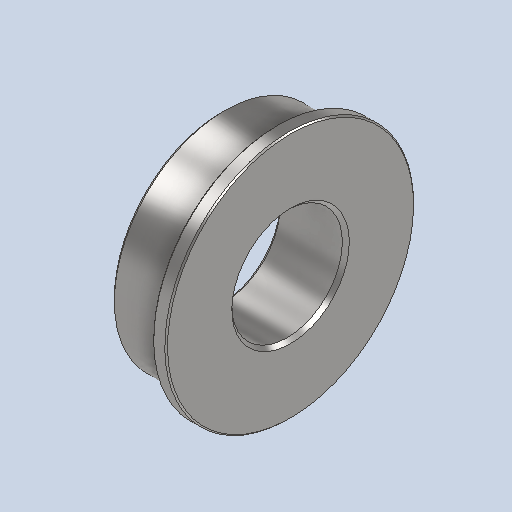
# Autodesk Inventor part: F688ZZ_V1
Saved by Autodesk Inventor 2023 (Build 270158000, 158)
## iProperties
Created: 2023-02-13
Part Number: F688ZZ_V1
Material: Stahl, Legierung
Document SubType Name: Modeling
Designer: Mathi
Density: 7.73 g/cm^3
Appearance: Halbpoliert
Author: Mathi
Autodesk Inventor part; units mm, degrees
ref_plane "YZ Plane" through (0, 0, 0) normal (1, 0, 0) x (0, 1, 0)
ref_plane "XZ Plane" through (0, 0, 0) normal (0, 1, 0) x (-1, 0, 0)
ref_plane "XY Plane" through (0, 0, 0) normal (0, 0, 1) x (1, 0, 0)
sketch "Skizze1" plane through (0, 0, 0) normal (0, 0, 1) x (1, 0, 0)
  line L0 (-18.8104, 0) -> (17.0467, 0)
  line L1 (-3.75, 4) -> (0.75, 4)
  line L2 (1, 4.25) -> (1, 8.9)
  line L3 (0.9, 9) -> (0.1, 9)
  line L4 (0, 8.9) -> (0, 8)
  line L5 (0, 8) -> (-3.75, 8)
  line L6 (-4, 7.75) -> (-4, 4.25)
  line L7 (-3.75, 8) -> (-4, 7.75)
  line L8 (-3.75, 4) -> (-4, 4.25)
  line L9 (0.75, 4) -> (1, 4.25)
  line L10 (0.1, 9) -> (0, 8.9)
  line L11 (1, 8.9) -> (0.9, 9)
  point P0 (0, 0)
  point P1 (-4, 4)
  point P2 (1, 4)
  point P3 (1, 9)
  point P4 (0, 9)
  point P5 (-4, 8)
  dimension "d0" = 5
  dimension "d1" = 18
  dimension "d2" = 1
  dimension "d3" = 16
  dimension "d4" = 8
  dimension "d5" = 0.25
  dimension "d6" = 0.25
  dimension "d7" = 0.25
  dimension "d8" = 0.25
  dimension "d9" = 0.25
  dimension "d10" = 0.25
  dimension "d11" = 0.1
  dimension "d12" = 0.1
  dimension "d13" = 0.1
  dimension "d14" = 0.1
  constraints: 24 end point, 12 point on line, 5 perpendicular, 2 horizontal
  measures "d0" distance between parallel lines of L2 L6
  measures "d1" diameter of L3 L0
  measures "d2" distance between parallel lines of L2 L4
  measures "d3" diameter of L5 L0
  measures "d4" diameter of L1 L0
  measures "d5" distance of L5.end point (-4, 8)
  measures "d6" distance of L6.start point (-4, 8)
  measures "d7" distance of L1.start point (-4, 4)
  measures "d8" distance of L6.end point (-4, 4)
  measures "d9" distance of L1.end point (1, 4)
  measures "d10" distance of L2.start point (1, 4)
  measures "d11" distance of L3.end point (0, 9)
  measures "d12" distance of L4.start point (0, 9)
  measures "d13" distance of L2.end point (1, 9)
  measures "d14" distance of L3.start point (1, 9)
revolve "Umdrehung1" add sketch "Skizze1" angle 360 about axis through (-18.8104, 0, 0) along (1, 0, 0)
equation "\"d6\" = d5"
equation "\"d7\" = d5"
equation "\"d8\" = d7"
equation "\"d9\" = d5"
equation "\"d10\" = d9"
equation "\"d12\" = d11"
equation "\"d14\" = d13"
